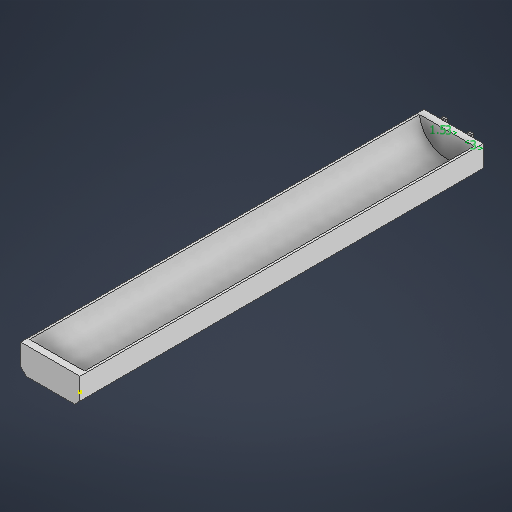
# Autodesk Inventor part: profilrampa
Saved by Autodesk Inventor 2026.2 (Build 302298000, 298)
## iProperties
Created: 2025-11-25
Part Number: profilrampa
Material: Generic
Document SubType Name: Modeling
Designer: janek
Density: 1 g/cm^3
Appearance: Default
Author: janek
Autodesk Inventor part; units mm, degrees
ref_plane "YZ Plane" through (0, 0, 0) normal (1, 0, 0) x (0, 1, 0)
ref_plane "XZ Plane" through (0, 0, 0) normal (0, 1, 0) x (-1, 0, 0)
ref_plane "XY Plane" through (0, 0, 0) normal (0, 0, 1) x (1, 0, 0)
sketch "Sketch1" plane through (0, 0, 0) normal (0, 1, 0) x (-1, 0, 0)
  line L0 (0, 0) -> (44, 0)
  line L1 (44, 0) -> (44, -300)
  line L2 (44, -300) -> (0, -300)
  line L3 (0, -300) -> (0, 0)
  dimension "d0" = 300
  dimension "d1" = 44
  constraints: 8 end point, 2 parallel, 1 horizontal, 1 perpendicular
  measures "d0" distance of L0.end L1.end
  measures "d1" distance between parallel lines of L3 L1
extrude "Extrusion1" add sketch "Sketch1" along normal blind 20
sketch "Sketch2" plane through (-44, 0, 0) normal (0, 0, 1) x (1, 0, 0)
  line L0 (44, 20) -> (0, 20) projected
  line L1 (44, 0) -> (0, 0) projected
  line L2 (0, 0) -> (44, 0)
  line L3 (44, 0) -> (44, 22)
  line L4 (44, 22) -> (0, 22)
  line L5 (0, 22) -> (0, 0)
  circle A0 centre (22, 22) radius 20.5
  dimension "d17" = 22
  dimension "d18" = 41
  dimension "d19" = 22
  constraints: 8 end point, 2 parallel, 1 centre point, 1 horizontal, 1 midpoint, 1 perpendicular
  measures "d17" distance of L2.end L3.end
  measures "d18" diameter of A0
  measures "d19" distance from line of L5 A0.centre
extrude "Extrusion2" cut sketch "Sketch2" against normal up to surface (300 mm away) contours A0 L0 | L0 A0 L4 | L4 A0
sketch "Sketch3" plane through (-44, 0, 0) normal (0, 0, 1) x (1, 0, 0)
  line L0 (0, 0) -> (0, 20) projected
  line L1 (0, 20) -> (44, 20)
  line L2 (44, 20) -> (44, 0)
  line L3 (44, 0) -> (0, 0)
  line L4 (0, 0) -> (0, 20)
  constraints: 8 end point, 2 parallel, 1 horizontal, 1 perpendicular
extrude "Extrusion3" add sketch "Sketch3" against normal blind 5
sketch "Sketch4" plane through (0, 0, -300) normal (0, 0, -1) x (-1, 0, 0)
  line L0 (0, 0) -> (0, 20) projected
  line L1 (44, 0) -> (0, 0) projected
  line L2 (0, 20) -> (44, 20)
  line L3 (44, 20) -> (44, 0)
  line L4 (44, 0) -> (0, 0)
  line L5 (0, 0) -> (0, 20)
  constraints: 8 end point, 2 parallel, 1 horizontal, 1 perpendicular
extrude "Extrusion4" add sketch "Sketch4" against normal blind 5
chamfer "Chamfer1" distance 4 angle 45 1 edges at (0, 0, -150)
chamfer "Chamfer2" distance 4 angle 45 1 edges at (-44, 0, -150)
sketch "Sketch5" plane through (0, 20, -300) normal (0, 0, -1) x (-1, 0, 0)
  line L0 (0, 0) -> (44, 0)
  line L1 (44, 0) -> (44, -20)
  line L2 (44, -20) -> (0, -20)
  line L3 (0, -20) -> (0, 0)
  line L4 (44, -16) -> (40, -20) projected
  line L5 (4, -20) -> (0, -16) projected
  line L6 (22, 0) -> (22, -20)
  line L7 (0, -10) -> (44, -10)
  line L8 (11.8539, 0) -> (11.8539, -20)
  line L9 (32.3539, 0) -> (32.3539, -20)
  line L10 (10.8539, 0) -> (10.8539, -20)
  line L11 (33.3539, 0) -> (33.3539, -20)
  line L12 (0, -9) -> (44, -9)
  circle A0 centre (11.8539, 0) radius 2
  circle A1 centre (32.3539, 0) radius 2
  point P0 (0, -20)
  point P1 (2, -18)
  point P2 (42, -18)
  point P3 (11.8539, -2)
  point P4 (10.8539, -1.7321)
  point P5 (10.8539, -10)
  point P6 (33.3539, -10)
  point P7 (33.3539, -1.7321)
  point P8 (32.3539, -2)
  point P9 (32.3539, -9)
  point P10 (11.8539, -9)
  dimension "d20" = 20
  dimension "d21" = 44
  dimension "d23" = 2
  dimension "d24" = 2
  dimension "d25" = 20.5
  dimension "d26" = 11.8539
  dimension "d27" = 1
  dimension "d28" = 1
  dimension "d29" = 9
  dimension "d30" = 4
  dimension "d31" = 4
  constraints: 20 end point, 6 point on line, 5 midpoint, 4 vertical, 2 centre point, 2 coincident, 2 horizontal, 2 perpendicular, 1 parallel, 8 other
  measures "d20" distance of L3.start L0.start
  measures "d21" distance between parallel lines of L1 L3
  measures "d23" horizontal distance of L3.start point (2, -18)
  measures "d24" horizontal distance of L1.end point (42, -18)
  measures "d25" distance between parallel lines of L9 L8
  measures "d26" distance between parallel lines of L3 L8
  measures "d27" distance between parallel lines of L10 L8
  measures "d28" distance between parallel lines of L9 L11
  measures "d29" distance between parallel lines of L12 L0
  measures "d30" diameter of A0
  measures "d31" diameter of A1
extrude "Extrusion5" add sketch "Sketch5" along normal blind 2.5 contours A0 L8 L12 L10 | L12 L8 L7 L10 | L12 L6 L7 L8 | L12 L9 L7 L6 | A1 L11 L12 L9 | L12 L11 L7 L9
sketch "Sketch7" plane through (-33.3539, 10, -300) normal (0, -1, 0) x (1, 0, 0)
  line L0 (22.5, -2.5) -> (0, -2.5)
  line L1 (0, -2.5) -> (0, -4)
  line L2 (0, -4) -> (22.5, -4)
  line L3 (22.5, -4) -> (22.5, -2.5)
  line L4 (0, 0) -> (0, -2.5) projected
  line L5 (22.5, -4) -> (21.5, -4)
  line L6 (21.5, -2.5) -> (22.5, -2.5)
  line L7 (22.5, -2.5) -> (22.5, -4)
  line L8 (21.5, 0) -> (21.5, -2.5) projected
  line L9 (3, -2.5) -> (0, -2.5)
  line L10 (0, -2.5) -> (0, -4)
  line L11 (0, -4) -> (3, -4)
  line L12 (3, -4) -> (3, -2.5)
  line L13 (22.5, -2.5) -> (0, -2.5) projected
  line L14 (22.5, -4) -> (19.5, -4)
  line L15 (19.5, -4) -> (19.5, -2.5)
  line L16 (19.5, -2.5) -> (22.5, -2.5)
  line L17 (22.5, -2.5) -> (22.5, -4)
  point P0 (33.3539, 300)
  point P1 (22.5, -3.25)
  point P2 (19.5, -4)
  point P3 (19.5, -2.5)
  point P4 (3, -4)
  dimension "d36" = 1.5
  dimension "d37" = 3
  dimension "d38" = 3
  constraints: 30 end point, 8 parallel, 4 horizontal, 3 perpendicular, 2 point on line, 1 collinear, 1 midpoint, 2 other
  measures "d36" distance between parallel lines of L0 L2
  measures "d37" distance from line of point (22.5, -3.25) L15
  measures "d38" distance between parallel lines of L12 L1
extrude "Extrusion6" add sketch "Sketch7" against normal blind 3 contours L15 L2 L12 L0
extrude "Extrusion7" add sketch "Sketch7" against normal blind 9 contours L3 L2 L15 L0 | L12 L2 L1 L0
body "Solid1"
